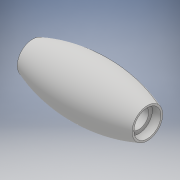
# Autodesk Inventor part: Roller 48mm
Saved by Autodesk Inventor 2018 (Build 220112000, 112)
## iProperties
Created: 2017-08-01
Part Number: Roller 48mm
Material: Generic
Document SubType Name: Modeling
Designer: P445885
Density: 1 g/cm^3
Appearance: Default
Author: P445885
Autodesk Inventor part; units mm, degrees
note: some values were not read from the file. Chosen so that the rebuilt part matches the saved one: direction of "Hole2".
ref_plane "YZ Plane" through (0, 0, 0) normal (1, 0, 0) x (0, 1, 0)
ref_plane "XZ Plane" through (0, 0, 0) normal (0, 1, 0) x (-1, 0, 0)
sketch "Sketch1" plane through (0, 0, 0) normal (0, 0, 1) x (1, 0, 0)
  circle A0 centre (0, 0) radius 100 construction
  circle A1 centre (0, 0) radius 75 construction
  circle A2 centre (0, 75) radius 25 construction
  circle A3 centre (0, 0) radius 89 construction
  dimension "d1" = 150
  dimension "d0" = 200
  dimension "d3" = 50
  dimension "d4" = 14
  constraints: 3 centre point, 2 coincident, 2 vertical alignment, 2 other
  measures "d0" diameter of A0
  measures "d3" diameter of A2
ref_plane "Work Plane1" through (0, 0, 0) normal (0, -0.7071068, 0.7071068) x (1, 0, 0)
sketch "Sketch2" plane through (0, 0, 0) normal (0, -0.7071068, 0.7071068) x (1, 0, 0)
  ellipse E0 centre (0, 0) end of major axis (100, 0) minor radius 70.7107 construction
  circle A0 centre (0, 45.7107) radius 25 construction
  circle A1 centre (0, 45.7107) radius 22 construction
  circle A2 centre (0, 45.7107) radius 12.5 construction
  line L0 (0, 58.2107) -> (46.793, 58.2107) construction
  line L1 (46.793, 45.7107) -> (-46.793, 45.7107)
  line L2 (0, 45.7107) -> (0, 58.2107) construction
  line L3 (0, 58.2107) -> (-46.793, 58.2107) construction
  ellipse E1 centre (0, 0) end of major axis (-96.8498, 0) minor radius 67.7107 (49.4713, 58.2107) -> (-49.4713, 58.2107) ccw construction
  line L4 (-46.793, 58.2107) -> (-46.793, 45.7107)
  line L5 (46.793, 58.2107) -> (46.793, 45.7107)
  circle A3 centre (0, 45.7107) radius 21 construction
  spline S0 degree 5 poles (103, 0) (102.9997, 6.0067) (102.15, 12.0166) (100.4439, 17.8567) (95.335, 29.4916) (87.5543, 39.5637) (82.9111, 44.3403) (72.1684, 53.435) (59.9286, 60.4121) (53.1788, 63.5338) (38.7726, 68.8984) (23.7279, 72.0795) (15.8518, 73.167) (0.0001, 74.2544) (-15.8515, 73.167) (-23.7275, 72.0796) (-38.7724, 68.8985) (-53.1787, 63.534) (-59.9287, 60.4119) (-72.1688, 53.435) (-82.9115, 44.3398) (-87.5547, 39.5637) (-95.3351, 29.4907) (-100.4441, 17.8572) (-102.1497, 12.015) (-103.8502, 0) (-102.1497, -12.015) (-100.4441, -17.8572) (-95.3351, -29.4907) (-87.5547, -39.5637) (-82.9115, -44.3398) (-72.1688, -53.435) (-59.9287, -60.4119) (-53.1787, -63.534) (-38.7724, -68.8985) (-23.7275, -72.0796) (-15.8515, -73.167) (0.0001, -74.2544) (15.8518, -73.167) (23.7279, -72.0795) (38.7726, -68.8984) (53.1788, -63.5338) (59.9286, -60.4121) (72.1684, -53.435) (82.9111, -44.3403) (87.5543, -39.5637) (95.335, -29.4916) (100.4439, -17.8567) (102.15, -12.0166) (102.9997, -6.0067) (103, 0) knots 0 0 0 0 0 0 0.053721 0.053721 0.053721 0.112881 0.112881 0.112881 0.179119 0.179119 0.179119 0.25 0.25 0.25 0.320879 0.320879 0.320879 0.38712 0.38712 0.38712 0.44628 0.44628 0.44628 0.5 0.5 0.5 0.55372 0.55372 0.55372 0.61288 0.61288 0.61288 0.679121 0.679121 0.679121 0.75 0.75 0.75 0.820881 0.820881 0.820881 0.887119 0.887119 0.887119 0.946279 0.946279 0.946279 1 1 1 1 1 1 construction
  spline S1 degree 5 poles (125, 0) (124.9996, 8.8962) (123.6824, 17.7961) (121.0383, 26.425) (113.3824, 42.8537) (101.833, 56.8343) (95.2127, 63.1614) (80.4494, 74.6213) (63.7738, 83.0792) (54.8985, 86.6443) (36.372, 92.4116) (17.1764, 95.263) (7.3437, 95.9828) (-12.2502, 95.9826) (-31.6302, 93.1025) (-41.1422, 90.9507) (-59.3601, 85.2856) (-76.3656, 76.6479) (-84.2872, 71.6905) (-98.7984, 60.4396) (-110.4889, 46.2955) (-115.3769, 38.6773) (-122.9533, 22.3258) (-125.6666, 4.5154) (-125.6666, -4.5154) (-122.9533, -22.3258) (-115.3769, -38.6773) (-110.4889, -46.2955) (-98.7984, -60.4396) (-84.2872, -71.6905) (-76.3656, -76.6479) (-59.3601, -85.2856) (-41.1422, -90.9507) (-31.6302, -93.1025) (-12.2502, -95.9826) (7.3437, -95.9828) (17.1764, -95.263) (36.372, -92.4116) (54.8985, -86.6443) (63.7738, -83.0792) (80.4494, -74.6213) (95.2127, -63.1614) (101.833, -56.8343) (113.3824, -42.8537) (121.0383, -26.425) (123.6824, -17.7961) (124.9996, -8.8962) (125, 0) knots 0 0 0 0 0 0 0.063791 0.063791 0.063791 0.128941 0.128941 0.128941 0.197218 0.197218 0.197218 0.267663 0.267663 0.267663 0.337325 0.337325 0.337325 0.403955 0.403955 0.403955 0.468142 0.468142 0.468142 0.531858 0.531858 0.531858 0.596045 0.596045 0.596045 0.662675 0.662675 0.662675 0.732337 0.732337 0.732337 0.802782 0.802782 0.802782 0.871059 0.871059 0.871059 0.936209 0.936209 0.936209 1 1 1 1 1 1 construction
  spline S2 degree 5 poles (46.793, 58.2107) (42.0231, 60.0696) (37.1481, 61.6587) (32.1958, 62.9892) (18.4817, 65.9465) (4.4646, 67.0684) (-4.4646, 67.0684) (-18.4817, 65.9465) (-32.1958, 62.9892) (-37.1481, 61.6587) (-42.0231, 60.0696) (-46.793, 58.2107) knots 0 0 0 0 0 0 0.267579 0.267579 0.267579 0.732421 0.732421 0.732421 1 1 1 1 1 1
  point P0 (0, 53.033)
  point P1 (0, 53.033)
  dimension "d17" = 3
  dimension "d28" = 25
  dimension "d25" = 50
  dimension "d27" = 3
  dimension "d29" = 9.5
  dimension "d50" = 46.793
  dimension "d51" = 46.793
  dimension "d52" = 1
  constraints: 12 end point, 5 horizontal, 3 centre point, 3 coincident, 2 perpendicular, 2 point on line, 2 vertical alignment, 1 horizontal alignment, 1 midpoint, 1 vertical, 15 other
  measures "d25" diameter of A0
  measures "d27" radial gap between concentric circles of A0 A1
  measures "d50" distance between parallel lines of L2 L5
  measures "d51" distance from line of point (0, 53.033) L5
  measures "d52" radial gap between concentric circles of A1 A3
revolve "Revolution1" add sketch "Sketch2" angle 360 about axis through (46.793, 32.3223, 32.3223) along (-1, 0, 0)
sketch "Sketch5" plane through (-46.793, 32.3223, 32.3223) normal (-1, 0, 0) x (0, 0, 1)
  circle A0 centre (0, 0) radius 12.5 projected
  circle A1 centre (0, 0) radius 11
  point P0 (-32.3223, -32.3223)
  point P1 (8.8388, 8.8388)
  dimension "d53" = 22
  constraints: 1 centre point, 1 coincident, 1 other
  measures "d53" diameter of A1
extrude "Extrusion3" cut sketch "Sketch5" against normal blind 7 contours A1
sketch "Sketch6" plane through (46.793, 32.3223, 32.3223) normal (1, 0, 0) x (0, 0, -1)
  circle A0 centre (0, 0) radius 12.5 projected
  circle A1 centre (0, 0) radius 11
  point P0 (32.3223, -32.3223)
  point P1 (-8.8388, 8.8388)
  dimension "d56" = 22
  constraints: 1 centre point, 1 coincident, 1 other
  measures "d56" diameter of A1
extrude "Extrusion4" cut sketch "Sketch6" against normal blind 7 contours A1
hole "Hole2" at (-39.793, 32.3223, 32.3223) direction (1, 0, 0) diameter 16 end up to surface
body "Solid1"
